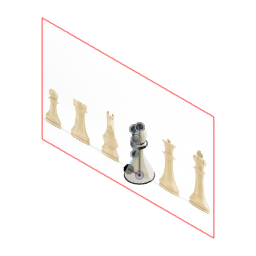
Board v4 (Autodesk Fusion 360 archive; units mm, degrees)
design "Bishop"
Autodesk Fusion 360 part; units mm, degrees
sketch "Sketch1" plane through (0, 0, 0) normal (0, 1, 0) x (1, 0, 0)
  line L0 (0, 0) -> (0, -80)
  line L1 (0, 0) -> (-20, 0)
  line L2 (-6.0501, -55.2545) -> (-10.2637, -52.2049)
  line L3 (-10.4525, -50.8951) -> (-5.4129, -45.8555)
  line L4 (-10.2637, -52.2049) -> (-10.4525, -50.8951)
  line L5 (0, -70.5202) -> (-2.9993, -80)
  line L6 (-2.9993, -80) -> (0, -80)
  spline S0 degree 5 poles (-20, 0) (-20, -0.6734) (-19.8627, -2.1332) (-19.2448, -4.6616) (-17.6673, -8.6584) (-14.8349, -14.4044) (-11.653, -20.5245) (-8.6578, -26.6258) (-6.3321, -32.3545) (-5.0054, -37.4666) (-4.7896, -41.8717) (-5.5103, -44.8202) (-6.5359, -46.7178) (-7.4317, -47.8457) (-7.9327, -48.3753) knots 0 0 0 0 0 0 0.1 0.2 0.3 0.4 0.5 0.6 0.7 0.8 0.9 1 1 1 1 1 1
  spline S1 degree 5 poles (-6.6133, -54.8469) (-6.9485, -55.5323) (-7.579, -56.8841) (-8.4052, -58.855) (-9.2635, -61.3672) (-9.9029, -64.3011) (-10.0667, -67.0089) (-9.7113, -69.4697) (-8.8041, -71.6681) (-7.3543, -73.6084) (-5.3976, -75.3076) (-3.4574, -76.4886) (-1.8044, -77.2803) (-0.6159, -77.767) (0, -78) knots 0 0 0 0 0 0 0.1 0.2 0.3 0.4 0.5 0.6 0.7 0.8 0.9 1 1 1 1 1 1
  line L7 (-20, 3) -> (-20, -3)
  point P0 (-7, -31)
  point P1 (-9.3943, -69.9909)
  dimension "d2" = 20
  dimension "d5" = 80
  dimension "d7" = 45
  constraint coincident L0.start L1.start
  constraint vertical L0
  constraint perpendicular L0 L1
  constraint coincident L0 L5.start
  constraint perpendicular L0 L6
  constraint coincident L0.end L6.end
  constraint coincident L3 S0.end
  constraint midpoint L3 S0.end
  constraint coincident L2 S1.start
  constraint coincident L0 S1.end
  constraint midpoint L1.end L7
  measures "d2" distance of L0.start L1.end
  measures "d5" distance of L0.start L0.end
  measures "d7" angle of L0 L3
revolve "Revolve1" add sketch "Sketch1" angle 360 about axis through (0, 0, 0) along (0, 0, 1)
sketch "Sketch2" plane through (0, 0, 0) normal (0, 1, 0) x (1, 0, 0)
  line L0 (-5.5, -78) -> (-0.7405, -62.5113)
  line L1 (-0.7405, -62.5113) -> (1.027, -63.0544)
  line L2 (1.027, -63.0544) -> (-3.8706, -78.9928)
  arc A0 (1.027, -63.0544) -> (-0.7405, -62.5113) centre (0.1432, -62.7828) ccw
  line L3 (-5.5, -78) -> (-3.8706, -78.9928)
  constraint perpendicular L0 L1
  constraint perpendicular L1 L2
extrude "Extrude1" cut sketch "Sketch2" along normal through all and the other way through all
equation "d1 = 8 cm"
equation "d2 = d1 * 1 / 4"

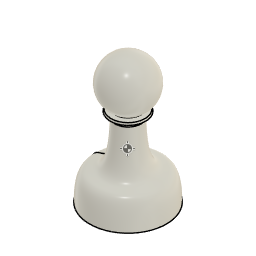
design "Pawn"
Autodesk Fusion 360 part; units mm, degrees
sketch "Sketch1" plane through (0, 0, 0) normal (0, 1, 0) x (1, 0, 0)
  line L0 (0, 0) -> (-15, 0)
  spline S0 degree 5 poles (-15, 0) (-15, -2.4594) (-14.7958, -6.5576) (-13.8775, -10.2456) (-11.6701, -11.3146) (-8.3299, -11.1548) (-6.1225, -14.3711) (-5.2042, -21.1026) (-5, -27.9377) (-5, -31.9428) knots 0 0 0 0 0 0 0.2 0.4 0.6 0.8 1 1 1 1 1 1
  line L1 (-15, 5) -> (-15, -5)
  line L2 (0, 0) -> (0, -50)
  line L3 (-5, -23.8005) -> (-5, -40.085)
  line L4 (-5, -31.9428) -> (-6.6248, -31.4797)
  line L5 (-6.9086, -30.7495) -> (-5.0265, -28.8674)
  arc A0 (0, -30.5583) -> (0, -50) centre (0, -40.2791) ccw
  line L6 (-6.6248, -31.4797) -> (-6.9086, -30.7495)
  dimension "d2" = 15
  dimension "d4" = 50
  dimension "d5" = 45
  dimension "d10" = 5
  constraint coincident L0.start L2.start
  constraint horizontal L0
  constraint midpoint L0.end L1
  constraint vertical L1
  constraint perpendicular L0 L2
  constraint midpoint S0.end L3
  constraint vertical L3
  constraint coincident S0 L4.start
  constraint coincident S0 L5.end
  constraint coincident L2 A0.start
  constraint coincident L2 A0.centre
  constraint coincident S0.end A0
  constraint coincident L3 S0.end
  measures "d2" distance of L0.start L0.end
  measures "d4" distance of L0.start L2.end
  measures "d5" angle of L3 L5
  measures "d10" distance of L2 L3
revolve "Revolve1" add sketch "Sketch1" angle 360 about axis through (0, 0, 0) along (0, 0, 1)
equation "d2 = 1 / 2 * 3 cm"

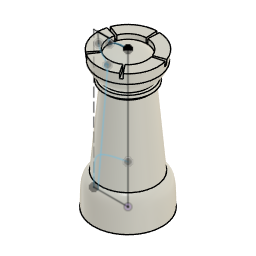
design "Rook"
Autodesk Fusion 360 part; units mm, degrees
sketch "Sketch1" plane through (0, 0, 0) normal (0, 1, 0) x (1, 0, 0)
  line L0 (0, 0) -> (0, -70)
  line L1 (0, 0) -> (-17.5, 0)
  spline S0 degree 5 poles (-17.5, 0) (-17.5, -1.949) (-17.4812, -5.4749) (-17.3967, -9.6483) (-17.034, -13.32) (-15.2217, -16.0242) (-11.5143, -17.5778) (-6.6893, -18.7492) (-2.4074, -19.5755) (0, -20) knots 0 0 0 0 0 0 0.2 0.4 0.6 0.8 1 1 1 1 1 1
  line L2 (-5, -19.1184) -> (5, -20.8816)
  line L3 (-17.5, 4) -> (-17.5, -4)
  line L4 (-15.4223, 0) -> (-10.3547, -57.9233)
  spline S1 degree 5 poles (-10.3547, -57.9233) (-10.6938, -58.2624) (-11.3394, -58.9222) (-12.2103, -59.8566) (-13.1936, -61.0089) (-14.1589, -62.3571) (-14.7035, -63.4078) (-14.9524, -64.1982) (-15.0388, -64.7286) (-15.0621, -64.9946) knots 0 0 0 0 0 0 0.2 0.4 0.6 0.8 1 1 1 1 1 1
  line L5 (-15.0621, -64.9946) -> (-15.5, -70)
  line L6 (-14.9783, -64.0369) -> (-15.1459, -65.9522)
  line L7 (-17.5, -70) -> (0, -70) construction
  line L8 (-15.5, -70) -> (-9.7348, -70)
  line L9 (-9.7348, -70) -> (-9.7348, -67.5)
  line L10 (-9.0716, -56.6402) -> (-11.6378, -59.2064)
  line L11 (-17.5, 0) -> (-17.5, -70) construction
  spline S2 degree 5 poles (-9.7348, -67.5) (-9.5938, -67.5) (-9.3202, -67.5511) (-8.9352, -67.7806) (-8.3991, -68.3325) (-7.2315, -69.1675) (-5.359, -69.7194) (-3.0799, -69.9489) (-1.103, -70) (0, -70) knots 0 0 0 0 0 0 0.2 0.4 0.6 0.8 1 1 1 1 1 1
  line L12 (-10.1589, -67.5) -> (-9.3107, -67.5)
  line L13 (-3.3162, -70) -> (3.3162, -70)
  line L14 (-10.3504, -57.9716) -> (-11.575, -57.6845)
  line L15 (-12.1293, -56.3884) -> (-10.6186, -54.9071)
  line L16 (-11.575, -57.6845) -> (-12.1293, -56.3884)
  dimension "d1" = 70
  dimension "d2" = 17.5
  dimension "d3" = 5
  dimension "d4" = 45
  dimension "d5" = 5
  dimension "d6" = 10
  dimension "d14" = 2.5
  dimension "d15" = 2
  constraint coincident L0.start L1.start
  constraint vertical L0
  constraint perpendicular L0 L1
  constraint midpoint L2 S0.end
  constraint midpoint L1.end L3
  constraint vertical L3
  constraint midpoint S1.end L6
  constraint parallel L5 L6
  constraint coincident L7 L8.end
  constraint perpendicular L8 L9
  constraint midpoint L4.end L10
  constraint vertical L11
  constraint horizontal L7
  constraint coincident L0 S0.end
  constraint coincident L1 L4.start
  constraint midpoint L9.end L12
  constraint perpendicular L9 L12
  constraint midpoint L0.end L13
  constraint perpendicular L0 L13
  constraint perpendicular L7 L9
  constraint coincident L4 L14.start
  constraint coincident L4 L15.end
  measures "d1" distance of L0.start L0.end
  measures "d2" distance of L0.start L1.end
  measures "d3" angle of L0 L5
  measures "d4" angle of L0 L10
  measures "d5" angle of L0 L4
  measures "d6" angle of L1 L2
  measures "d14" distance of L8.end L9.end
  measures "d15" distance of L5.end L7.start
revolve "Revolve1" add sketch "Sketch1" angle 360 about axis through (0, 0, 0) along (0, 0, 1)
sketch "Sketch3" plane through (0, 0, 70) normal (0, 0, 1) x (-1, 0, 0)
  circle A0 centre (0, 0) radius 9.7348
  circle A1 centre (0, 0) radius 15.5
  line L0 (0, 0) -> (0.6761, -15.4852)
  line L1 (0, 0) -> (-0.6761, -15.4852)
  line L2 (0, 0) -> (0, -15.5) construction
  dimension "d8" = 5
  dimension "d9" = 2.5
  constraint coincident A0.centre A1.centre
  constraint coincident A1 L0.end
  constraint coincident A1 L1.end
  constraint coincident A1 L2.end
  measures "d8" angle of L0 L1
  measures "d9" angle of L1 L2
extrude "Extrude1" cut sketch "Sketch3" against normal up to surface (2.5 mm away) contours A0 A1 L0 L1 picked at (0.4421, -13.5697)
pattern_circular "C-Pattern1" count 5 over 360 about axis through (0, 0, 1.75) along (0, 0, 1) of "Extrude1"
equation "d2 = 3.5 cm / 2"

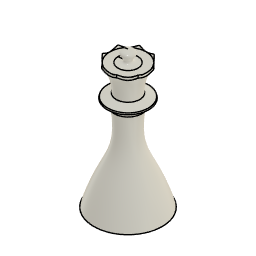
design "Queen"
Autodesk Fusion 360 part; units mm, degrees
sketch "Sketch1" plane through (0, 0, 0) normal (0, 1, 0) x (1, 0, 0)
  line L0 (0, 0) -> (0, -85)
  line L1 (0, 0) -> (-21.25, 0)
  spline S0 degree 5 poles (-21.25, 0) (-20.5462, -2.3433) (-19.1499, -6.7502) (-17.0895, -12.5209) (-14.4454, -18.6826) (-11.5056, -24.6083) (-9.1582, -29.6604) (-7.603, -34.6438) (-6.9084, -39.9689) (-6.9734, -45.5239) (-7.2538, -50.0318) (-7.6365, -52.5133) (-8.0931, -53.7597) (-8.4928, -54.335) (-8.7164, -54.5586) knots 0 0 0 0 0 0 0.1 0.2 0.3 0.4 0.5 0.6 0.7 0.8 0.9 1 1 1 1 1 1
  line L2 (-7.02, -37.2676) -> (-6.98, -48.7324)
  line L3 (-24.4738, 10.7337) -> (-18.0262, -10.7337)
  line L4 (-12.8771, -58.7193) -> (-8.7164, -54.5586)
  line L5 (-12.638, -59.5462) -> (-12.8771, -58.7193)
  line L6 (-7.343, -61.5169) -> (-12.638, -59.5462)
  line L7 (-6.8181, -52.6603) -> (-10.6147, -56.4569)
  spline S1 degree 5 poles (-13.1569, -78.5027) (-12.4892, -77.7088) (-11.2807, -76.1544) (-9.8487, -73.923) (-8.5957, -71.1204) (-7.7576, -67.8087) (-7.4445, -65.2532) (-7.3447, -63.3722) (-7.3342, -62.1329) (-7.343, -61.5169) knots 0 0 0 0 0 0 0.2 0.4 0.6 0.8 1 1 1 1 1 1
  line L8 (-14.6843, -80.3185) -> (-11.6296, -76.6868)
  line L9 (-13.1569, -78.5027) -> (-12.3917, -79.1464)
  line L10 (-11.3516, -77.8444) -> (0, -77.8444)
  spline S2 degree 3 poles (-12.3917, -79.1464) (-12.0221, -78.707) (-11.676, -78.2731) (-11.3516, -77.8444) knots 0 0 0 0 0.067818 0.067818 0.067818 0.067818
  spline S3 degree 5 poles (0, -85) (-0.2704, -85) (-0.7932, -84.9807) (-1.5236, -84.8938) (-2.3815, -84.6694) (-3.2166, -84.2487) (-3.7573, -83.7253) (-3.9628, -83.1299) (-3.7936, -82.4359) (-3.3163, -81.6293) (-2.7424, -80.7887) (-2.2901, -79.9992) (-2.1518, -79.3422) (-2.3237, -78.8165) (-2.7541, -78.3928) (-3.493, -78.0775) (-4.3771, -77.9184) (-5.2343, -77.8579) (-5.8959, -77.8444) (-6.2493, -77.8444) knots 0 0 0 0 0 0 0.066667 0.133333 0.2 0.266667 0.333333 0.4 0.466667 0.533333 0.6 0.666667 0.733333 0.8 0.866667 0.933333 1 1 1 1 1 1
  line L11 (-3.9297, -77.8444) -> (-8.5689, -77.8444)
  line L12 (-2.2286, -80.1018) -> (-2.2286, -78.7046)
  line L13 (-3.8706, -83.8443) -> (-3.8706, -82.2964)
  line L14 (1.7404, -85) -> (-1.7404, -85)
  point P0 (-7, -43)
  point P1 (-3.8706, -83.0703)
  point P2 (-2.2286, -79.4032)
  dimension "d1" = 85
  dimension "d2" = 21.25
  dimension "d3" = 45
  constraint coincident L0.start L1.start
  constraint vertical L0
  constraint perpendicular L0 L1
  constraint midpoint P0 L2
  constraint midpoint L1.end L3
  constraint midpoint S0.end L7
  constraint parallel L4 L7
  constraint midpoint S1.start L8
  constraint coincident L0 L10.end
  constraint perpendicular L0 L10
  constraint coincident L10 S3.end
  constraint midpoint S3.end L11
  constraint parallel L10 L11
  constraint midpoint P2 L12
  constraint parallel L0 L12
  constraint midpoint P1 L13
  constraint parallel L0 L13
  constraint midpoint L0.end L14
  constraint perpendicular L0 L14
  measures "d1" distance of L0.start L0.end
  measures "d2" distance of L0.start L1.end
  measures "d3" angle of L0 L4
revolve "Revolve1" add sketch "Sketch1" angle 360 about axis through (0, 0, 0) along (0, 0, 1)
sketch "Sketch3" plane through (0, 0, 0) normal (0, 0, 1) x (1, 0, 0)
  line L0 (0, 0) -> (0, 11.3516) construction
  line L1 (0, 11.3516) -> (0, 13.1569) construction
  circle A0 centre (0, 0) radius 13.1569
  circle A1 centre (0, 0) radius 11.3516 construction
  spline S0 degree 5 poles (-8.242, 10.2554) (-7.917, 10.5166) (-7.2759, 10.9649) (-6.3405, 11.4151) (-5.1187, 11.6257) (-3.4944, 11.5235) (-1.6638, 11.3506) (0.4217, 11.3289) (2.5464, 11.4125) (4.5486, 11.4203) (6.3999, 11.1591) (7.7699, 10.5717) (8.7526, 9.8467) (9.3907, 9.2269) (9.7056, 8.883) knots 0 0 0 0 0 0 0.1 0.2 0.3 0.4 0.5 0.6 0.7 0.8 0.9 1 1 1 1 1 1
  line L2 (9.368, 9.2518) -> (10.0431, 8.5141)
  line L3 (-8.6318, 9.9422) -> (-7.8523, 10.5686)
  line L4 (-0.5, 11.3511) -> (0.5, 11.3521)
  dimension "d9" = 18
  dimension "d12" = 1
  dimension "d13" = 1
  constraint coincident L0.start A0.centre
  constraint vertical L0
  constraint parallel L0 L1
  constraint coincident L1.end A0
  constraint coincident L0.end A1
  constraint coincident A0 S0.start
  constraint coincident A0 S0.end
  constraint midpoint S0.end L2
  constraint tangent A0 L2
  constraint midpoint S0.start L3
  constraint tangent A0 L3
  constraint midpoint L0.end L4
  constraint tangent A1 L4
  constraint equal L2 L3
  measures "d9" distance of S0.start S0.end
  measures "d12" distance of L2.start L2.end
  measures "d13" horizontal distance of L4.start L4.end
extrude "Extrude1" cut sketch "Sketch3" along normal blind 10 from surface at 75 contours A0 S0 picked at (0.7318, 11.832)
pattern_circular "C-Pattern1" count 8 over 360 about axis through (0, 0, 1.75) along (0, 0, 1) of "Extrude1"
equation "d2 = 1 / 4 * d1"
